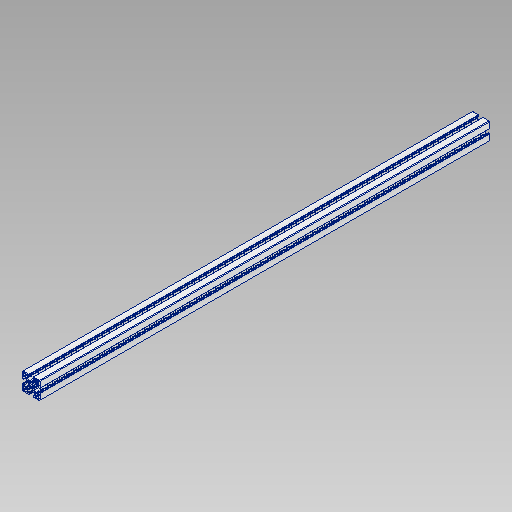
# Autodesk Inventor part: dnf3030_720
Saved by Autodesk Inventor 2026.2 (Build 302298000, 298)
## iProperties
Created: 2026-02-25
Part Number: dnf3030_720
Material: 알루미늄 6061
Document SubType Name: Modeling
Designer: mjbhang
Density: 2.7 g/cm^3
Appearance: 알루미늄 - 평지
Author: mjbhang
Autodesk Inventor part; units mm, degrees
ref_plane "YZ Plane" through (0, 0, 0) normal (1, 0, 0) x (0, 1, 0)
ref_plane "XZ Plane" through (0, 0, 0) normal (0, 1, 0) x (-1, 0, 0)
ref_plane "XY Plane" through (0, 0, 0) normal (0, 0, 1) x (1, 0, 0)
sketch "스케치1" plane through (0, 0, 0) normal (0, 0, 1) x (1, 0, 0)
  line L0 (3.9512, -15.0012) -> (3.1512, -14.5012)
  line L1 (3.1512, -14.5012) -> (3.1512, -12.8012)
  arc A0 (3.4512, -12.5012) -> (3.1512, -12.8012) centre (3.4512, -12.8012) ccw
  line L2 (3.4512, -12.5012) -> (5.1012, -12.5012)
  line L3 (5.1012, -12.5012) -> (6.0888, -9.4494)
  arc A1 (6.0888, -9.4494) -> (6.1145, -8.929) centre (5.1374, -9.1415) ccw
  arc A2 (6.1145, -8.929) -> (4.0052, -5.0909) centre (-3.3582, -11.6363) ccw
  arc A3 (4.0052, -5.0909) -> (2.219, -4.5012) centre (2.219, -7.5012) ccw
  line L4 (2.219, -4.5012) -> (0.5012, -4.5012)
  line L5 (0.5012, -4.5012) -> (0.0012, -4.0012)
  line L6 (0.0012, -4.0012) -> (-0.4988, -4.5012)
  line L7 (-0.4988, -4.5012) -> (-2.2167, -4.5012)
  arc A4 (-2.2167, -4.5012) -> (-4.0028, -5.0909) centre (-2.2167, -7.5012) ccw
  arc A5 (-4.0028, -5.0909) -> (-6.1122, -8.929) centre (3.3606, -11.6363) ccw
  arc A6 (-6.1122, -8.929) -> (-6.0864, -9.4494) centre (-5.135, -9.1415) ccw
  line L8 (-6.0864, -9.4494) -> (-5.0988, -12.5012)
  line L9 (-5.0988, -12.5012) -> (-3.4488, -12.5012)
  arc A7 (-3.1488, -12.8012) -> (-3.4488, -12.5012) centre (-3.4488, -12.8012) ccw
  line L10 (-3.1488, -12.8012) -> (-3.1488, -14.5012)
  line L11 (-3.1488, -14.5012) -> (-3.9488, -15.0012)
  line L12 (-3.9488, -15.0012) -> (-13.9988, -15.0012)
  arc A8 (-14.9988, -14.0012) -> (-13.9988, -15.0012) centre (-13.9988, -14.0012) ccw
  line L13 (-14.9988, -14.0012) -> (-14.9988, -3.9512)
  line L14 (-14.9988, -3.9512) -> (-14.4988, -3.1512)
  line L15 (-14.4988, -3.1512) -> (-12.7988, -3.1512)
  arc A9 (-12.4988, -3.4512) -> (-12.7988, -3.1512) centre (-12.7988, -3.4512) ccw
  line L16 (-12.4988, -3.4512) -> (-12.4988, -5.1012)
  line L17 (-12.4988, -5.1012) -> (-9.4471, -6.0888)
  arc A10 (-9.4471, -6.0888) -> (-8.9267, -6.1145) centre (-9.1392, -5.1374) ccw
  arc A11 (-8.9267, -6.1145) -> (-5.0885, -4.0052) centre (-11.6339, 3.3582) ccw
  arc A12 (-5.0885, -4.0052) -> (-4.4988, -2.219) centre (-7.4988, -2.219) ccw
  line L18 (-4.4988, -2.219) -> (-4.4988, -0.5012)
  line L19 (-4.4988, -0.5012) -> (-3.9988, -0.0012)
  line L20 (-3.9988, -0.0012) -> (-4.4988, 0.4988)
  line L21 (-4.4988, 0.4988) -> (-4.4988, 2.2167)
  arc A13 (-4.4988, 2.2167) -> (-5.0885, 4.0028) centre (-7.4988, 2.2167) ccw
  arc A14 (-5.0885, 4.0028) -> (-8.9267, 6.1122) centre (-11.6339, -3.3606) ccw
  arc A15 (-8.9267, 6.1122) -> (-9.4471, 6.0864) centre (-9.1392, 5.135) ccw
  line L22 (-9.4471, 6.0864) -> (-12.4988, 5.0988)
  line L23 (-12.4988, 5.0988) -> (-12.4988, 3.4488)
  arc A16 (-12.7988, 3.1488) -> (-12.4988, 3.4488) centre (-12.7988, 3.4488) ccw
  line L24 (-12.7988, 3.1488) -> (-14.4988, 3.1488)
  line L25 (-14.4988, 3.1488) -> (-14.9988, 3.9488)
  line L26 (-14.9988, 3.9488) -> (-14.9988, 13.9988)
  arc A17 (-13.9988, 14.9988) -> (-14.9988, 13.9988) centre (-13.9988, 13.9988) ccw
  line L27 (-13.9988, 14.9988) -> (-3.9488, 14.9988)
  line L28 (-3.9488, 14.9988) -> (-3.1488, 14.4988)
  line L29 (-3.1488, 14.4988) -> (-3.1488, 12.7988)
  arc A18 (-3.4488, 12.4988) -> (-3.1488, 12.7988) centre (-3.4488, 12.7988) ccw
  line L30 (-3.4488, 12.4988) -> (-5.0988, 12.4988)
  line L31 (-5.0988, 12.4988) -> (-6.0864, 9.4471)
  arc A19 (-6.0864, 9.4471) -> (-6.1122, 8.9267) centre (-5.135, 9.1392) ccw
  arc A20 (-6.1122, 8.9267) -> (-4.0028, 5.0885) centre (3.3606, 11.6339) ccw
  arc A21 (-4.0028, 5.0885) -> (-2.2167, 4.4988) centre (-2.2167, 7.4988) ccw
  line L32 (-2.2167, 4.4988) -> (-0.4988, 4.4988)
  line L33 (-0.4988, 4.4988) -> (0.0012, 3.9988)
  line L34 (0.0012, 3.9988) -> (0.5012, 4.4988)
  line L35 (0.5012, 4.4988) -> (2.219, 4.4988)
  arc A22 (2.219, 4.4988) -> (4.0052, 5.0885) centre (2.219, 7.4988) ccw
  arc A23 (4.0052, 5.0885) -> (6.1145, 8.9267) centre (-3.3582, 11.6339) ccw
  arc A24 (6.1145, 8.9267) -> (6.0888, 9.4471) centre (5.1374, 9.1392) ccw
  line L36 (6.0888, 9.4471) -> (5.1012, 12.4988)
  line L37 (5.1012, 12.4988) -> (3.4512, 12.4988)
  arc A25 (3.1512, 12.7988) -> (3.4512, 12.4988) centre (3.4512, 12.7988) ccw
  line L38 (3.1512, 12.7988) -> (3.1512, 14.4988)
  line L39 (3.1512, 14.4988) -> (3.9512, 14.9988)
  line L40 (3.9512, 14.9988) -> (14.0012, 14.9988)
  arc A26 (15.0012, 13.9988) -> (14.0012, 14.9988) centre (14.0012, 13.9988) ccw
  line L41 (15.0012, 13.9988) -> (15.0012, 3.9488)
  line L42 (15.0012, 3.9488) -> (14.5012, 3.1488)
  line L43 (14.5012, 3.1488) -> (12.8012, 3.1488)
  arc A27 (12.5012, 3.4488) -> (12.8012, 3.1488) centre (12.8012, 3.4488) ccw
  line L44 (12.5012, 3.4488) -> (12.5012, 5.0988)
  line L45 (12.5012, 5.0988) -> (9.4494, 6.0864)
  arc A28 (9.4494, 6.0864) -> (8.929, 6.1122) centre (9.1415, 5.135) ccw
  arc A29 (8.929, 6.1122) -> (5.0909, 4.0028) centre (11.6363, -3.3606) ccw
  arc A30 (5.0909, 4.0028) -> (4.5012, 2.2167) centre (7.5012, 2.2167) ccw
  line L46 (4.5012, 2.2167) -> (4.5012, 0.4988)
  line L47 (4.5012, 0.4988) -> (4.0012, -0.0012)
  line L48 (4.0012, -0.0012) -> (4.5012, -0.5012)
  line L49 (4.5012, -0.5012) -> (4.5012, -2.219)
  arc A31 (4.5012, -2.219) -> (5.0909, -4.0052) centre (7.5012, -2.219) ccw
  arc A32 (5.0909, -4.0052) -> (8.929, -6.1145) centre (11.6363, 3.3582) ccw
  arc A33 (8.929, -6.1145) -> (9.4494, -6.0888) centre (9.1415, -5.1374) ccw
  line L50 (9.4494, -6.0888) -> (12.5012, -5.1012)
  line L51 (12.5012, -5.1012) -> (12.5012, -3.4512)
  arc A34 (12.8012, -3.1512) -> (12.5012, -3.4512) centre (12.8012, -3.4512) ccw
  line L52 (12.8012, -3.1512) -> (14.5012, -3.1512)
  line L53 (14.5012, -3.1512) -> (15.0012, -3.9512)
  line L54 (15.0012, -3.9512) -> (15.0012, -14.0012)
  arc A35 (14.0012, -15.0012) -> (15.0012, -14.0012) centre (14.0012, -14.0012) ccw
  line L55 (14.0012, -15.0012) -> (3.9512, -15.0012)
  arc A36 (7.3121, -8.6656) -> (7.2557, -8.3199) centre (7.0435, -8.532) ccw
  line L56 (7.2557, -8.3199) -> (6.5152, -7.5793)
  arc A37 (6.4937, -7.1789) -> (6.5152, -7.5793) centre (6.7273, -7.3671) ccw
  arc A38 (7.1756, -6.4971) -> (6.4937, -7.1789) centre (9.9981, -10.0019) ccw
  arc A39 (7.5759, -6.5187) -> (7.1756, -6.4971) centre (7.3638, -6.7308) ccw
  line L57 (7.5759, -6.5187) -> (8.3164, -7.2593)
  arc A40 (8.3164, -7.2593) -> (8.6622, -7.3158) centre (8.5286, -7.0472) ccw
  arc A41 (11.3344, -7.316) -> (8.6622, -7.3158) centre (9.9981, -10.0019) ccw
  arc A42 (11.3344, -7.316) -> (11.6801, -7.2596) centre (11.468, -7.0474) ccw
  line L58 (11.6801, -7.2596) -> (12.4207, -6.5191)
  arc A43 (12.8211, -6.4976) -> (12.4207, -6.5191) centre (12.6329, -6.7312) ccw
  arc A44 (13.5029, -7.1795) -> (12.8211, -6.4976) centre (9.9981, -10.0019) ccw
  arc A45 (13.4813, -7.5798) -> (13.5029, -7.1795) centre (13.2692, -7.3677) ccw
  line L59 (13.4813, -7.5798) -> (12.7407, -8.3203)
  arc A46 (12.7407, -8.3203) -> (12.6842, -8.6661) centre (12.9528, -8.5325) ccw
  arc A47 (12.684, -11.3383) -> (12.6842, -8.6661) centre (9.9981, -10.0019) ccw
  arc A48 (12.684, -11.3383) -> (12.7404, -11.684) centre (12.9526, -11.4719) ccw
  line L60 (12.7404, -11.684) -> (13.4809, -12.4246)
  arc A49 (13.5024, -12.825) -> (13.4809, -12.4246) centre (13.2688, -12.6368) ccw
  arc A50 (12.8205, -13.5068) -> (13.5024, -12.825) centre (9.9981, -10.0019) ccw
  arc A51 (12.4202, -13.4852) -> (12.8205, -13.5068) centre (12.6323, -13.2731) ccw
  line L61 (12.4202, -13.4852) -> (11.6797, -12.7446)
  arc A52 (11.6797, -12.7446) -> (11.3339, -12.6881) centre (11.4675, -12.9567) ccw
  arc A53 (8.6617, -12.6879) -> (11.3339, -12.6881) centre (9.9981, -10.0019) ccw
  arc A54 (8.6617, -12.6879) -> (8.316, -12.7443) centre (8.5281, -12.9565) ccw
  line L62 (8.316, -12.7443) -> (7.5754, -13.4848)
  arc A55 (7.175, -13.5063) -> (7.5754, -13.4848) centre (7.3632, -13.2727) ccw
  arc A56 (6.4932, -12.8244) -> (7.175, -13.5063) centre (9.9981, -10.0019) ccw
  arc A57 (6.5148, -12.4241) -> (6.4932, -12.8244) centre (6.7269, -12.6362) ccw
  line L63 (6.5148, -12.4241) -> (7.2554, -11.6836)
  arc A58 (7.2554, -11.6836) -> (7.3119, -11.3378) centre (7.0433, -11.4714) ccw
  arc A59 (7.3121, -8.6656) -> (7.3119, -11.3378) centre (9.9981, -10.0019) ccw
  line L64 (7.7981, -10.0018) -> (12.1981, -10.0021)
  line L65 (9.9982, -7.8019) -> (9.9979, -12.2019)
  arc A60 (3.2385, 1.585) -> (3.4436, 2.0328) centre (3.1853, 1.8802) ccw
  arc A61 (3.4436, 2.0328) -> (2.0352, 3.4412) centre (0, -0.0023) ccw
  arc A62 (2.0352, 3.4412) -> (1.5873, 3.2362) centre (1.8825, 3.1829) ccw
  line L66 (1.5873, 3.2362) -> (1.4537, 2.4952)
  arc A63 (1.0345, 2.2753) -> (1.4537, 2.4952) centre (1.1585, 2.5485) ccw
  arc A64 (1.0345, 2.2753) -> (-1.0321, 2.2753) centre (0.0012, -0.0012) ccw
  arc A65 (-1.4514, 2.4952) -> (-1.0321, 2.2753) centre (-1.1561, 2.5485) ccw
  line L67 (-1.4514, 2.4952) -> (-1.585, 3.2362)
  arc A66 (-1.585, 3.2362) -> (-2.0328, 3.4412) centre (-1.8802, 3.1829) ccw
  arc A67 (-2.0328, 3.4412) -> (-3.4412, 2.0328) centre (0.0023, -0.0023) ccw
  arc A68 (-3.4412, 2.0328) -> (-3.2362, 1.585) centre (-3.1829, 1.8802) ccw
  line L68 (-3.2362, 1.585) -> (-2.4952, 1.4514)
  arc A69 (-2.2753, 1.0321) -> (-2.4952, 1.4514) centre (-2.5485, 1.1561) ccw
  arc A70 (-2.2753, 1.0321) -> (-2.2753, -1.0345) centre (0.0012, -0.0012) ccw
  arc A71 (-2.4952, -1.4537) -> (-2.2753, -1.0345) centre (-2.5485, -1.1585) ccw
  line L69 (-2.4952, -1.4537) -> (-3.2362, -1.5873)
  arc A72 (-3.2362, -1.5873) -> (-3.4412, -2.0352) centre (-3.1829, -1.8825) ccw
  arc A73 (-3.4412, -2.0352) -> (-2.0328, -3.4436) centre (0.0023, 0) ccw
  arc A74 (-2.0328, -3.4436) -> (-1.585, -3.2385) centre (-1.8802, -3.1853) ccw
  line L70 (-1.585, -3.2385) -> (-1.4514, -2.4976)
  arc A75 (-1.0321, -2.2776) -> (-1.4514, -2.4976) centre (-1.1561, -2.5508) ccw
  arc A76 (-1.0321, -2.2776) -> (1.0345, -2.2776) centre (0.0012, -0.0012) ccw
  arc A77 (1.4537, -2.4976) -> (1.0345, -2.2776) centre (1.1585, -2.5508) ccw
  line L71 (1.4537, -2.4976) -> (1.5873, -3.2385)
  arc A78 (1.5873, -3.2385) -> (2.0352, -3.4436) centre (1.8825, -3.1853) ccw
  arc A79 (2.0352, -3.4436) -> (3.4436, -2.0352) centre (0, 0) ccw
  arc A80 (3.4436, -2.0352) -> (3.2385, -1.5873) centre (3.1853, -1.8825) ccw
  line L72 (3.2385, -1.5873) -> (2.4976, -1.4537)
  arc A81 (2.2776, -1.0345) -> (2.4976, -1.4537) centre (2.5508, -1.1585) ccw
  arc A82 (2.2776, -1.0345) -> (2.2776, 1.0321) centre (0.0012, -0.0012) ccw
  arc A83 (2.4976, 1.4514) -> (2.2776, 1.0321) centre (2.5508, 1.1561) ccw
  line L73 (2.4976, 1.4514) -> (3.2385, 1.585)
  arc A84 (-7.3128, 8.6627) -> (-7.2563, 8.317) centre (-7.0442, 8.5291) ccw
  line L74 (-7.2563, 8.317) -> (-6.5157, 7.5764)
  arc A85 (-6.4942, 7.1761) -> (-6.5157, 7.5764) centre (-6.7279, 7.3643) ccw
  arc A86 (-7.1761, 6.4942) -> (-6.4942, 7.1761) centre (-9.9988, 9.9988) ccw
  arc A87 (-7.5764, 6.5157) -> (-7.1761, 6.4942) centre (-7.3643, 6.7279) ccw
  line L75 (-7.5764, 6.5157) -> (-8.317, 7.2563)
  arc A88 (-8.317, 7.2563) -> (-8.6627, 7.3128) centre (-8.5291, 7.0442) ccw
  arc A89 (-11.3349, 7.3128) -> (-8.6627, 7.3128) centre (-9.9988, 9.9988) ccw
  arc A90 (-11.3349, 7.3128) -> (-11.6807, 7.2563) centre (-11.4686, 7.0442) ccw
  line L76 (-11.6807, 7.2563) -> (-12.4213, 6.5157)
  arc A91 (-12.8216, 6.4942) -> (-12.4213, 6.5157) centre (-12.6334, 6.7279) ccw
  arc A92 (-13.5034, 7.1761) -> (-12.8216, 6.4942) centre (-9.9988, 9.9988) ccw
  arc A93 (-13.4819, 7.5764) -> (-13.5034, 7.1761) centre (-13.2698, 7.3643) ccw
  line L77 (-13.4819, 7.5764) -> (-12.7413, 8.317)
  arc A94 (-12.7413, 8.317) -> (-12.6849, 8.6627) centre (-12.9535, 8.5291) ccw
  arc A95 (-12.6849, 11.3349) -> (-12.6849, 8.6627) centre (-9.9988, 9.9988) ccw
  arc A96 (-12.6849, 11.3349) -> (-12.7413, 11.6807) centre (-12.9535, 11.4686) ccw
  line L78 (-12.7413, 11.6807) -> (-13.4819, 12.4213)
  arc A97 (-13.5034, 12.8216) -> (-13.4819, 12.4213) centre (-13.2698, 12.6334) ccw
  arc A98 (-12.8216, 13.5034) -> (-13.5034, 12.8216) centre (-9.9988, 9.9988) ccw
  arc A99 (-12.4213, 13.4819) -> (-12.8216, 13.5034) centre (-12.6334, 13.2698) ccw
  line L79 (-12.4213, 13.4819) -> (-11.6807, 12.7413)
  arc A100 (-11.6807, 12.7413) -> (-11.3349, 12.6849) centre (-11.4686, 12.9535) ccw
  arc A101 (-8.6627, 12.6849) -> (-11.3349, 12.6849) centre (-9.9988, 9.9988) ccw
  arc A102 (-8.6627, 12.6849) -> (-8.317, 12.7413) centre (-8.5291, 12.9535) ccw
  line L80 (-8.317, 12.7413) -> (-7.5764, 13.4819)
  arc A103 (-7.1761, 13.5034) -> (-7.5764, 13.4819) centre (-7.3643, 13.2698) ccw
  arc A104 (-6.4942, 12.8216) -> (-7.1761, 13.5034) centre (-9.9988, 9.9988) ccw
  arc A105 (-6.5157, 12.4213) -> (-6.4942, 12.8216) centre (-6.7279, 12.6334) ccw
  line L81 (-6.5157, 12.4213) -> (-7.2563, 11.6807)
  arc A106 (-7.2563, 11.6807) -> (-7.3128, 11.3349) centre (-7.0442, 11.4686) ccw
  arc A107 (-7.3128, 8.6627) -> (-7.3128, 11.3349) centre (-9.9988, 9.9988) ccw
  arc A108 (7.2563, 8.317) -> (7.3128, 8.6627) centre (7.0442, 8.5291) ccw
  line L82 (7.2563, 8.317) -> (6.5157, 7.5764)
  arc A109 (6.5157, 7.5764) -> (6.4942, 7.1761) centre (6.7279, 7.3643) ccw
  arc A110 (6.4942, 7.1761) -> (7.1761, 6.4942) centre (9.9988, 9.9988) ccw
  arc A111 (7.1761, 6.4942) -> (7.5764, 6.5157) centre (7.3643, 6.7279) ccw
  line L83 (7.5764, 6.5157) -> (8.317, 7.2563)
  arc A112 (8.6627, 7.3128) -> (8.317, 7.2563) centre (8.5291, 7.0442) ccw
  arc A113 (8.6627, 7.3128) -> (11.3349, 7.3128) centre (9.9988, 9.9988) ccw
  arc A114 (11.6807, 7.2563) -> (11.3349, 7.3128) centre (11.4686, 7.0442) ccw
  line L84 (11.6807, 7.2563) -> (12.4213, 6.5157)
  arc A115 (12.4213, 6.5157) -> (12.8216, 6.4942) centre (12.6334, 6.7279) ccw
  arc A116 (12.8216, 6.4942) -> (13.5034, 7.1761) centre (9.9988, 9.9988) ccw
  arc A117 (13.5034, 7.1761) -> (13.4819, 7.5764) centre (13.2698, 7.3643) ccw
  line L85 (13.4819, 7.5764) -> (12.7413, 8.317)
  arc A118 (12.6849, 8.6627) -> (12.7413, 8.317) centre (12.9535, 8.5291) ccw
  arc A119 (12.6849, 8.6627) -> (12.6849, 11.3349) centre (9.9988, 9.9988) ccw
  arc A120 (12.7413, 11.6807) -> (12.6849, 11.3349) centre (12.9535, 11.4686) ccw
  line L86 (12.7413, 11.6807) -> (13.4819, 12.4213)
  arc A121 (13.4819, 12.4213) -> (13.5034, 12.8216) centre (13.2698, 12.6334) ccw
  arc A122 (13.5034, 12.8216) -> (12.8216, 13.5034) centre (9.9988, 9.9988) ccw
  arc A123 (12.8216, 13.5034) -> (12.4213, 13.4819) centre (12.6334, 13.2698) ccw
  line L87 (12.4213, 13.4819) -> (11.6807, 12.7413)
  arc A124 (11.3349, 12.6849) -> (11.6807, 12.7413) centre (11.4686, 12.9535) ccw
  arc A125 (11.3349, 12.6849) -> (8.6627, 12.6849) centre (9.9988, 9.9988) ccw
  arc A126 (8.317, 12.7413) -> (8.6627, 12.6849) centre (8.5291, 12.9535) ccw
  line L88 (8.317, 12.7413) -> (7.5764, 13.4819)
  arc A127 (7.5764, 13.4819) -> (7.1761, 13.5034) centre (7.3643, 13.2698) ccw
  arc A128 (7.1761, 13.5034) -> (6.4942, 12.8216) centre (9.9988, 9.9988) ccw
  arc A129 (6.4942, 12.8216) -> (6.5157, 12.4213) centre (6.7279, 12.6334) ccw
  line L89 (6.5157, 12.4213) -> (7.2563, 11.6807)
  arc A130 (7.3128, 11.3349) -> (7.2563, 11.6807) centre (7.0442, 11.4686) ccw
  arc A131 (7.3128, 11.3349) -> (7.3128, 8.6627) centre (9.9988, 9.9988) ccw
  line L90 (-9.9988, 7.7988) -> (-9.9988, 12.1988)
  line L91 (-7.7988, 9.9988) -> (-12.1988, 9.9988)
  line L92 (7.7988, 9.9988) -> (12.1988, 9.9988)
  line L93 (9.9988, 7.7988) -> (9.9988, 12.1988)
  line L94 (0.0012, -15.9423) -> (0.0012, 15.9951)
  line L95 (15.4588, -0.0012) -> (-16.223, -0.0012)
  arc A132 (-7.2557, -8.3199) -> (-7.3121, -8.6656) centre (-7.0435, -8.532) ccw
  line L96 (-7.2557, -8.3199) -> (-6.5152, -7.5793)
  arc A133 (-6.5152, -7.5793) -> (-6.4937, -7.1789) centre (-6.7273, -7.3671) ccw
  arc A134 (-6.4937, -7.1789) -> (-7.1756, -6.4971) centre (-9.9981, -10.0019) ccw
  arc A135 (-7.1756, -6.4971) -> (-7.5759, -6.5187) centre (-7.3638, -6.7308) ccw
  line L97 (-7.5759, -6.5187) -> (-8.3164, -7.2593)
  arc A136 (-8.6622, -7.3158) -> (-8.3164, -7.2593) centre (-8.5286, -7.0472) ccw
  arc A137 (-8.6622, -7.3158) -> (-11.3344, -7.316) centre (-9.9981, -10.0019) ccw
  arc A138 (-11.6801, -7.2596) -> (-11.3344, -7.316) centre (-11.468, -7.0474) ccw
  line L98 (-11.6801, -7.2596) -> (-12.4207, -6.5191)
  arc A139 (-12.4207, -6.5191) -> (-12.8211, -6.4976) centre (-12.6329, -6.7312) ccw
  arc A140 (-12.8211, -6.4976) -> (-13.5029, -7.1795) centre (-9.9981, -10.0019) ccw
  arc A141 (-13.5029, -7.1795) -> (-13.4813, -7.5798) centre (-13.2692, -7.3677) ccw
  line L99 (-13.4813, -7.5798) -> (-12.7407, -8.3203)
  arc A142 (-12.6842, -8.6661) -> (-12.7407, -8.3203) centre (-12.9528, -8.5325) ccw
  arc A143 (-12.6842, -8.6661) -> (-12.684, -11.3383) centre (-9.9981, -10.0019) ccw
  arc A144 (-12.7404, -11.684) -> (-12.684, -11.3383) centre (-12.9526, -11.4719) ccw
  line L100 (-12.7404, -11.684) -> (-13.4809, -12.4246)
  arc A145 (-13.4809, -12.4246) -> (-13.5024, -12.825) centre (-13.2688, -12.6368) ccw
  arc A146 (-13.5024, -12.825) -> (-12.8205, -13.5068) centre (-9.9981, -10.0019) ccw
  arc A147 (-12.8205, -13.5068) -> (-12.4202, -13.4852) centre (-12.6323, -13.2731) ccw
  line L101 (-12.4202, -13.4852) -> (-11.6797, -12.7446)
  arc A148 (-11.3339, -12.6881) -> (-11.6797, -12.7446) centre (-11.4675, -12.9567) ccw
  arc A149 (-11.3339, -12.6881) -> (-8.6617, -12.6879) centre (-9.9981, -10.0019) ccw
  arc A150 (-8.316, -12.7443) -> (-8.6617, -12.6879) centre (-8.5281, -12.9565) ccw
  line L102 (-8.316, -12.7443) -> (-7.5754, -13.4848)
  arc A151 (-7.5754, -13.4848) -> (-7.175, -13.5063) centre (-7.3632, -13.2727) ccw
  arc A152 (-7.175, -13.5063) -> (-6.4932, -12.8244) centre (-9.9981, -10.0019) ccw
  arc A153 (-6.4932, -12.8244) -> (-6.5148, -12.4241) centre (-6.7269, -12.6362) ccw
  line L103 (-6.5148, -12.4241) -> (-7.2554, -11.6836)
  arc A154 (-7.3119, -11.3378) -> (-7.2554, -11.6836) centre (-7.0433, -11.4714) ccw
  arc A155 (-7.3119, -11.3378) -> (-7.3121, -8.6656) centre (-9.9981, -10.0019) ccw
  line L104 (-7.7981, -10.0018) -> (-12.1981, -10.0021)
  line L105 (-9.9982, -7.8019) -> (-9.9979, -12.2019)
  point P0 (0, 0)
  constraints: 312 point on circle, 212 end point, 156 centre point, 4 point on line
extrude "돌출1" add sketch "스케치1" against normal blind 770 contours L0 L1 A0 L2 L3 A1 A2 A3 L4 L5 L94 A76 A77 L71 A78 A79 A80 L72 A81 A82 L95 L48 L49 A31 A32 A33 L50 L51 A34 L52 L53 L54 A35 L55 | L6 L7 A4 A5 A6 L8 L9 A7 L10 L11 L12 A8 L13 L14 L15 A9 L16 L17 A10 A11 A12 L18 L19 L95 A70 A71 L69 A72 A73 A74 L70 A75 A76 L94 | L94 L34 L35 A22 A23 A24 L36 L37 A25 L38 L39 L40 A26 L41 L42 L43 A27 L44 L45 A28 A29 A30 L46 L47 L95 A82 A83 L73 A60 A61 A62 L66 A63 A64 | A64 A65 L67 A66 A67 A68 L68 A69 A70 L95 L20 L21 A13 A14 A15 L22 L23 A16 L24 L25 L26 A17 L27 L28 L29 A18 L30 L31 A19 A20 A21 L32 L33 L94
